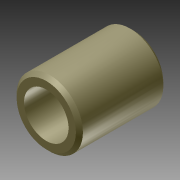
# Autodesk Inventor part: D-25359
Saved by Autodesk Inventor 2012 (Build 160160000, 160)
## iProperties
Created: 2013-01-17
Part Number: D-25359
Material: Default
Catalog Web Link: www.cadenas.de
Description: Bushing-Original Line - Standard Air Cylinders
Vendor: BIMBA
Document SubType Name: Modeling
Designer: William
Manufacturer: BIMBA
Density: 1 g/cm^3
Category: PARTsolutions
Company: BIMBA
Title: D-25359
Author: Cadenas PARTsolutions
Comments: Original Line - Standard Air Cylinders
PSOL_IDENT_0: {\\10.0.0.242\data_v9\23d-libs\bimba\bimba\bimba_imperial\bimba_full_line\original_line_cylinders\st
PSOL_IDENT_1: andard_air_cylinders\bushing.prj},157 {VTYP=3D},{NB=D-25359},{LINA=D-25359},{NN=Bushing},{DATE=13.09
PSOL_IDENT_2: .2012 05:23:39},{GEOMDATE=10.09.2012 00:00:00},{VERSION=},{LINEID=10},{LINESUBID=-1},{WBVAR=}  {NB=D
PSOL_IDENT_3: -25359},{LINA=D-25359},{KT=DUMMY},{PN=D-25359},{ID=0.1275},{OD=0.1895},{L=0.2500},{C=0.0100}
CNS_NT: Original Line - Standard Air Cylinders
CNS_NB: D-25359
CNS_NBSYN: $PN.
CNS_LINA: D-25359
CNS_PN: D-25359
CNS_ID: 0.1275
CNS_OD: 0.1895
CNS_L: 0.2500
CNS_C: 0.0100
SUPPLIER: BIMBA
ARTICLENO: D-25359
BOMINFO: D-25359
CREATOR: CADENAS GmbH
Autodesk Inventor part; units mm, degrees
sketch "Sketch_1" plane through (0, 0, 0) normal (1, 0, 0) x (0, 1, 0)
  line L0 (0, -3.175) -> (0, 3.175)
  line L1 (2.1526, 3.175) -> (1.6193, 3.175)
  line L2 (1.6193, 3.175) -> (1.6193, -3.175)
  line L3 (1.6193, -3.175) -> (2.1526, -3.175)
  line L4 (2.1526, -3.175) -> (2.4066, -2.921)
  line L5 (2.4066, -2.921) -> (2.4066, 2.921)
  line L6 (2.4066, 2.921) -> (2.1526, 3.175)
  constraints: 14 end point
revolve "Revolution1" add sketch "Sketch_1" angle 360 about axis through (0, 0, -3.175) along (0, 0, -1)
ref_plane "bushing_XY" through (0, 0, 0) normal (0, 0, 1) x (1, 0, 0)
ref_plane "bushing_YZ" through (0, 0, 0) normal (1, 0, 0) x (0, 1, 0)
ref_plane "bushing_ZX" through (0, 0, 0) normal (0, 1, 0) x (0, 0, 1)
ref_plane "id1_XY" through (-1.6193, 0, 0) normal (0, 0, 1) x (1, 0, 0)
ref_plane "id1_YZ" through (-1.6193, 0, 0) normal (1, 0, 0) x (0, 1, 0)
ref_plane "id1_ZX" through (-1.6193, 0, 0) normal (0, 1, 0) x (0, 0, 1)
ref_plane "id2_XY" through (1.6193, 0, 0) normal (0, 0, 1) x (1, 0, 0)
ref_plane "id2_YZ" through (1.6193, 0, 0) normal (1, 0, 0) x (0, 1, 0)
ref_plane "id2_ZX" through (1.6193, 0, 0) normal (0, 1, 0) x (0, 0, 1)
ref_plane "id3_XY" through (0, 0, -3.175) normal (0, 0, -1) x (0, 1, 0)
ref_plane "id3_YZ" through (0, 0, -3.175) normal (0, 1, 0) x (1, 0, 0)
ref_plane "id3_ZX" through (0, 0, -3.175) normal (1, 0, 0) x (0, 0, -1)
ref_plane "id4_XY" through (0, 0, 3.175) normal (0, 0, 1) x (0, 1, 0)
ref_plane "id4_YZ" through (0, 0, 3.175) normal (0, 1, 0) x (-1, 0, 0)
ref_plane "id4_ZX" through (0, 0, 3.175) normal (-1, 0, 0) x (0, 0, 1)
body "Solid1"
